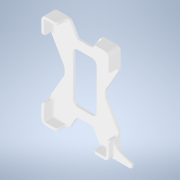
# Autodesk Inventor part: Heatpad Tray
Saved by Autodesk Inventor 2020 (Build 240168000, 168)
## iProperties
Created: 2020-02-13
Part Number: Heatpad Tray
Material: ABS Plastic
Document SubType Name: Modeling
Designer: Ishaan
Density: 1.06 g/cm^3
Appearance: Smooth - White
Author: Ishaan
Autodesk Inventor part; units mm, degrees
ref_plane "YZ Plane" through (0, 0, 0) normal (1, 0, 0) x (0, 1, 0)
sketch "Sketch1" plane through (0, 0, 0) normal (0, 0, 1) x (1, 0, 0)
  line L0 (38, -53) -> (-38, -53)
  line L1 (-38, -53) -> (-38, 53)
  line L2 (-38, 53) -> (38, 53)
  line L3 (38, 53) -> (38, -53)
  line L4 (38, -53) -> (-38, 53) construction
  line L5 (-38, -53) -> (38, 53) construction
  point P0 (0, 0)
  dimension "d0" = 76
  dimension "d1" = 106
  constraints: 12 end point, 2 midpoint, 2 parallel, 1 horizontal, 1 perpendicular
  measures "d0" distance of L1.end L2.end
  measures "d1" distance of L0.end L1.end
extrude "Extrusion1" add sketch "Sketch1" against normal blind 3
sketch "Sketch2" plane through (0, 0, 0) normal (0, 0, 1) x (1, 0, 0)
  line L0 (38, -53) -> (38, 53) projected
  line L1 (38, 53) -> (-38, 53) projected
  line L2 (-38, 53) -> (-38, -53) projected
  line L3 (-38, -53) -> (38, -53) projected
  line L4 (-35, -50) -> (-35, 50)
  line L5 (-35, 50) -> (35, 50)
  line L6 (35, 50) -> (35, -50)
  line L7 (35, -50) -> (-35, -50)
  line L8 (38, -53) -> (-38, -53) projected
  line L9 (20.5, 53) -> (-20.5, 53)
  line L10 (-20.5, 53) -> (-20.5, -53)
  line L11 (-20.5, -53) -> (20.5, -53)
  line L12 (20.5, -53) -> (20.5, 53)
  line L13 (20.5, 53) -> (-20.5, -53) construction
  line L14 (-20.5, 53) -> (20.5, -53) construction
  line L15 (-38, -53) -> (-38, 53) projected
  line L16 (38, 33) -> (-38, 33)
  line L17 (-38, 33) -> (-38, -33)
  line L18 (-38, -33) -> (38, -33)
  line L19 (38, -33) -> (38, 33)
  line L20 (38, 33) -> (-38, -33) construction
  line L21 (-38, 33) -> (38, -33) construction
  point P0 (0, 0)
  point P1 (35, -33)
  point P2 (20.5, -50)
  point P3 (20.5, -53)
  point P4 (35, 33)
  point P5 (20.5, 50)
  point P6 (-38, 33)
  point P7 (-35, 33)
  point P8 (-20.5, 50)
  point P9 (-20.5, 53)
  point P10 (-35, -33)
  point P11 (-20.5, -53)
  point P12 (-20.5, -50)
  dimension "d4" = 3
  dimension "d5" = 17.5
  dimension "d6" = 20
  constraints: 32 end point, 4 midpoint, 4 parallel, 2 horizontal, 2 perpendicular, 2 point on line, 3 other
  measures "d4" distance between parallel lines of L2 L4
  measures "d5" distance between parallel lines of L10 L2
  measures "d6" distance between parallel lines of L18 L3
extrude "Extrusion2" add sketch "Sketch2" along normal blind 11 contours L3 L12 L7 L6 L18 L0 | L16 L6 L5 L12 L1 L0 | L3 L2 L18 L4 L7 L10 | L10 L5 L4 L16 L2 L1
sketch "Sketch3" plane through (0, 0, 0) normal (0, 0, 1) x (1, 0, 0)
  line L0 (20.5, 50) -> (20.5, 53) projected
  line L1 (20.5, 53) -> (-20.5, 53) projected
  line L2 (-20.5, 53) -> (-20.5, 50) projected
  line L3 (-20.5, 50) -> (-35, 50) projected
  line L4 (-35, 50) -> (-35, 33) projected
  line L5 (-35, 33) -> (-38, 33) projected
  line L6 (-38, 33) -> (-38, -33) projected
  line L7 (-38, -33) -> (-35, -33) projected
  line L8 (-35, -33) -> (-35, -50) projected
  line L9 (-35, -50) -> (-20.5, -50) projected
  line L10 (-20.5, -50) -> (-20.5, -53) projected
  line L11 (-20.5, -53) -> (20.5, -53) projected
  line L12 (20.5, -53) -> (20.5, -50) projected
  line L13 (20.5, -50) -> (35, -50) projected
  line L14 (35, -50) -> (35, -33) projected
  line L15 (35, -33) -> (38, -33) projected
  line L16 (38, -33) -> (38, 33) projected
  line L17 (38, 33) -> (35, 33) projected
  line L18 (35, 33) -> (35, 50) projected
  line L19 (35, 50) -> (20.5, 50) projected
  line L20 (-38, 33) -> (-38, -33) projected
  line L21 (-38, -30) -> (-23, -4.0192)
  line L22 (-23, -4.0192) -> (-23, 0)
  line L23 (-20.5, -53) -> (20.5, -53) projected
  line L24 (-17.5, -53) -> (-8.8397, -38)
  line L25 (-8.8397, -38) -> (0, -38)
  line L26 (0, -38) -> (0, -53)
  line L27 (-23, 0) -> (-38, 0)
  point P0 (0, 0)
  dimension "d9" = 15
  dimension "d10" = 30
  dimension "d11" = 30
  dimension "d12" = 15
  dimension "d13" = 17.5
  constraints: 12 end point, 3 parallel, 2 midpoint, 2 perpendicular, 2 point on line
  measures "d9" distance between parallel lines of L22 L6
  measures "d10" angle of L6 L21
  measures "d11" distance of L21.start L27.end
  measures "d12" distance between parallel lines of L25 L11
  measures "d13" distance of L26.end L24.start
extrude "Extrusion3" cut sketch "Sketch3" against normal through all contours L27 L22 L21 L6 | L11 L24 L25 L26
mirror "Mirror1" about plane through (0, 0, 0) normal (1, 0, 0) of "Extrusion3"
mirror "Mirror2" about plane through (0, 0, 0) normal (0, 1, 0) of "Extrusion3", "Mirror1"
ref_plane "Work Plane1" through (0, 0, 4) normal (0, 0, -1) x (-1, 0, 0)
sketch "Sketch4" plane through (0, 0, 4) normal (0, 0, -1) x (-1, 0, 0)
  line L0 (-38, -33) -> (-35, -33) projected
  line L1 (-35, -33) -> (-35, -50) projected
  line L2 (-35, -50) -> (-20.5, -50) projected
  line L3 (-20.5, -50) -> (-20.5, -53) projected
  line L4 (-20.5, -53) -> (-38, -53) projected
  line L5 (-38, -53) -> (-38, -33) projected
  line L6 (-38, -53) -> (-17.5, -53) projected
  line L7 (-38, -53) -> (-58, -53)
  line L8 (-58, -53) -> (-58, -48)
  line L9 (-58, -48) -> (-38, -48)
  line L10 (-38, -48) -> (-38, -53)
  line L11 (-58, -48) -> (-38, -40.7206)
  line L12 (-38, -30) -> (-38, -53) projected
  line L13 (-38, -48) -> (-38, -40.7206)
  point P0 (0, 0)
  dimension "d16" = 20
  dimension "d17" = 5
  dimension "d30" = 70
  constraints: 12 end point, 2 parallel, 1 collinear, 1 horizontal, 1 perpendicular, 1 point on line
  measures "d16" distance of L8.end L9.end
  measures "d17" distance of L7.end L8.end
  measures "d30" angle of L11 L5
extrude "Extrusion4" add sketch "Sketch4" along normal mid plane 3 contours L5 L9 L11 | L5 L7 L8 L9
sketch "Sketch5" plane through (0, 0, 0) normal (0, 0, 1) x (1, 0, 0)
  line L0 (-13, -28) -> (13, -28)
  line L1 (13, -28) -> (13, 28)
  line L2 (13, 28) -> (-13, 28)
  line L3 (-13, 28) -> (-13, -28)
  line L4 (-13, -28) -> (13, 28) construction
  line L5 (13, -28) -> (-13, 28) construction
  line L6 (23, -4.0192) -> (23, 4.0192) projected
  line L7 (23, 4.0192) -> (38, 30) projected
  line L8 (38, 30) -> (38, 33) projected
  line L9 (38, 33) -> (35, 33) projected
  line L10 (35, 33) -> (35, 50) projected
  line L11 (35, 50) -> (20.5, 50) projected
  line L12 (20.5, 50) -> (20.5, 53) projected
  line L13 (20.5, 53) -> (17.5, 53) projected
  line L14 (17.5, 53) -> (8.8397, 38) projected
  line L15 (8.8397, 38) -> (-8.8397, 38) projected
  line L16 (-8.8397, 38) -> (-17.5, 53) projected
  line L17 (-17.5, 53) -> (-20.5, 53) projected
  line L18 (-20.5, 53) -> (-20.5, 50) projected
  line L19 (-20.5, 50) -> (-35, 50) projected
  line L20 (-35, 50) -> (-35, 33) projected
  line L21 (-35, 33) -> (-38, 33) projected
  line L22 (-38, 33) -> (-38, 30) projected
  line L23 (-38, 30) -> (-23, 4.0192) projected
  line L24 (-23, 4.0192) -> (-23, -4.0192) projected
  line L25 (-23, -4.0192) -> (-38, -30) projected
  line L26 (-38, -30) -> (-38, -33) projected
  line L27 (-38, -33) -> (-35, -33) projected
  line L28 (-35, -33) -> (-35, -50) projected
  line L29 (-35, -50) -> (-20.5, -50) projected
  line L30 (-20.5, -50) -> (-20.5, -53) projected
  line L31 (-20.5, -53) -> (-17.5, -53) projected
  line L32 (-17.5, -53) -> (-8.8397, -38) projected
  line L33 (-8.8397, -38) -> (8.8397, -38) projected
  line L34 (8.8397, -38) -> (17.5, -53) projected
  line L35 (17.5, -53) -> (20.5, -53) projected
  line L36 (20.5, -53) -> (20.5, -50) projected
  line L37 (20.5, -50) -> (35, -50) projected
  line L38 (35, -50) -> (35, -33) projected
  line L39 (35, -33) -> (38, -33) projected
  line L40 (38, -33) -> (38, -30) projected
  line L41 (38, -30) -> (23, -4.0192) projected
  point P0 (0, 0)
  dimension "d31" = 10
  dimension "d32" = 10
  constraints: 12 end point, 2 midpoint, 2 parallel, 1 horizontal, 1 perpendicular
  measures "d31" distance between parallel lines of L1 L6
  measures "d32" distance between parallel lines of L2 L15
extrude "Extrusion5" cut sketch "Sketch5" against normal through all contours L3 L2 L1 L0
fillet "Fillet1" radius 10 1 edges at (38, -40.7206, 4)
fillet "Fillet2" radius 2 2 edges at (58, -53, 4) (58, -48, 4)
fillet "Fillet3" radius 5 20 edges at (-17.5, -53, -1.5) (-8.8397, -38, -1.5) (17.5, -53, -1.5) (8.8397, -38, -1.5) (-17.5, 53, -1.5) (-8.8397, 38, -1.5) (8.8397, 38, -1.5) (17.5, 53, -1.5) (38, -30, -1.5) (23, -4.0192, -1.5) (23, 4.0192, -1.5) (38, 30, -1.5) (-38, -30, -1.5) (-23, -4.0192, -1.5) (-23, 4.0192, -1.5) (-38, 30, -1.5) (13, 28, -1.5) (-13, 28, -1.5) (13, -28, -1.5) (-13, -28, -1.5)
fillet "Fillet4" radius 3 16 edges at (-20.5, 51.5, 11) (-36.5, 33, 11) (-36.5, 33, 0) (-20.5, 51.5, 0) (20.5, 51.5, 11) (36.5, 33, 11) (36.5, 33, 0) (36.5, -33, 0) (36.5, -33, 11) (20.5, -51.5, 11) (20.5, -51.5, 0) (-20.5, -51.5, 0) (-20.5, -51.5, 11) (-36.5, -33, 11) (-36.5, -33, 0) (20.5, 51.5, 0)
fillet "Fillet5" radius 5 5 edges at (38, -53, 8.25) (38, -53, -0.25) (-38, -53, 4) (-38, 53, 4) (38, 53, 4)
fillet "Fillet6" radius 2 4 edges at (-35, -50, 5.5) (-35, 50, 5.5) (35, 50, 5.5) (35, -50, 5.5)
fillet "Fillet7" radius 2 20 edges at (-19, -50, 0) (-26.75, -50, 0) (-35, -31.5, 0) (-35, -40.5, 0) (-34.4142, -49.4142, 0) (-34.4142, 49.4142, 0) (-19, 50, 0) (-26.75, 50, 0) (-35, 40.5, 0) (-35, 31.5, 0) (34.4142, 49.4142, 0) (35, 40.5, 0) (35, 31.5, 0) (26.75, 50, 0) (19, 50, 0) (34.4142, -49.4142, 0) (35, -40.5, 0) (35, -31.5, 0) (26.75, -50, 0) (19, -50, 0)
fillet "Fillet8" radius 0.5 170 edges at (38, -33.8787, 10.1213) (38, -33, 5.5) (38, -32.5514, 1.4219) (37.9577, -30.6911, 0.0807) (37.6103, -29.4045, 0) (30.5, -17.0096, 0) (23.1704, -3.9736, 0) (23, 0, 0) (23.1704, 3.9736, 0) (30.5, 17.0096, 0) (37.6103, 29.4045, 0) (37.9577, 30.6911, 0.0807) (38, 32.5514, 1.4219) (38, 33, 5.5) (38, 33.8787, 10.1213) (38, 42, 11) (36.5355, 51.5355, 11) (28.25, 53, 11) (21.3787, 53, 10.1213) (20.5, 53, 5.5) (20.4716, 53, 2.5878) (19.3428, 52.8898, 0.6327) (16.6926, 51.3694, 0) (13.1699, 45.5, 0) (8.453, 38.6699, 0) (0, 38, 0) (-8.453, 38.6699, 0) (-13.1699, 45.5, 0) (-16.6926, 51.3694, 0) (-19.3428, 52.8898, 0.6327) (-20.4716, 53, 2.5878) (-20.5, 53, 5.5) (-21.3787, 53, 10.1213) (-28.25, 53, 11) (-36.5355, 51.5355, 11) (-38, 42, 11) (-38, 33.8787, 10.1213) (-38, 33, 5.5) (-38, 32.5514, 1.4219) (-37.9577, 30.6911, 0.0807) (-37.6103, 29.4045, 0) (-30.5, 17.0096, 0) (-23.1704, 3.9736, 0) (-23, 0, 0) (-23.1704, -3.9736, 0) (-30.5, -17.0096, 0) (-37.6103, -29.4045, 0) (-37.9577, -30.6911, 0.0807) (-38, -32.5514, 1.4219) (-38, -33, 5.5) (-38, -33.8787, 10.1213) (-38, -42, 11) (-36.5355, -51.5355, 11) (-28.25, -53, 11) (-21.3787, -53, 10.1213) (-20.5, -53, 5.5) (-20.4716, -53, 2.5878) (-19.3426, -52.8898, 0.6326) (-16.6926, -51.3694, 0) (-13.1699, -45.5, 0) (-8.453, -38.6699, 0) (0, -38, 0) (8.453, -38.6699, 0) (13.1699, -45.5, 0) (16.6926, -51.3694, 0) (19.3428, -52.8898, 0.6327) (20.4716, -53, 2.5878) (20.5, -53, 5.5) (21.3787, -53, 10.1213) (28.25, -53, 11) (36.5355, -51.5355, 11) (38, -42, 11) (34.4142, -49.4142, 11) (28.25, -50, 11) (21.3787, -50, 10.1213) (20.5, -50, 5.5) (20.4568, -50, 2.4927) (35, -33.8787, 10.1213) (35, -33, 5.5) (35, -32.9568, 2.4927) (35, -42, 11) (-28.25, -50, 11) (-34.4142, -49.4142, 11) (-35, -42, 11) (-35, -33.8787, 10.1213) (-35, -33, 5.5) (-35, -32.9568, 2.4927) (-34.2327, -31.5394, 0.4251) (-20.5, -50, 5.5) (-20.4568, -50, 2.4927) (-19.0394, -49.2327, 0.4251) (-21.3787, -50, 10.1213) (-35, 42, 11) (-34.4142, 49.4142, 11) (-28.25, 50, 11) (-21.3787, 50, 10.1213) (-20.5, 50, 5.5) (-20.4568, 50, 2.4927) (-19.0394, 49.2327, 0.4251) (-35, 33, 5.5) (-35, 32.9568, 2.4927) (-34.2327, 31.5394, 0.4251) (-35, 33.8787, 10.1213) (21.3787, 50, 10.1213) (28.25, 50, 11) (34.4142, 49.4142, 11) (35, 42, 11) (35, 33.8787, 10.1213) (35, 33, 5.5) (35, 32.9568, 2.4927) (34.2327, 31.5394, 0.4251) (20.4568, 50, 2.4927) (19.0394, 49.2327, 0.4251) (20.5, 50, 5.5) (-13.1699, 45.5, -3) (-17.8868, 52.3301, -3) (-26.6934, 53, -3) (-36.5355, 51.5355, -3) (-38, 39.6699, -3) (-37.8296, 30.0457, -3) (-30.5, 17.0096, -3) (-23.1704, 3.9736, -3) (-23, 0, -3) (-23.1704, -3.9736, -3) (-30.5, -17.0096, -3) (-37.8296, -30.0457, -3) (-38, -39.6699, -3) (-36.5355, -51.5355, -3) (-26.6934, -53, -3) (-17.8868, -52.3301, -3) (-13.1699, -45.5, -3) (-8.453, -38.6699, -3) (0, -38, -3) (8.453, -38.6699, -3) (13.1699, -45.5, -3) (17.8868, -52.3301, -3) (26.6934, -53, -3) (36.5355, -51.5355, -3) (38, -39.6699, -3) (37.8296, -30.0457, -3) (30.5, -17.0096, -3) (23.1704, -3.9736, -3) (23, 0, -3) (23.1704, 3.9736, -3) (30.5, 17.0096, -3) (37.8296, 30.0457, -3) (38, 39.6699, -3) (36.5355, 51.5355, -3) (26.6934, 53, -3) (17.8868, 52.3301, -3) (13.1699, 45.5, -3) (8.453, 38.6699, -3) (0, 38, -3) (-8.453, 38.6699, -3) (13, 0, -3) (11.5355, -26.5355, -3) (0, -28, -3) (-11.5355, -26.5355, -3) (-13, 0, -3) (-11.5355, 26.5355, -3) (0, 28, -3) (11.5355, 26.5355, -3) (0, 28, 0) (-11.5355, 26.5355, 0) (-13, 0, 0) (-11.5355, -26.5355, 0) (0, -28, 0) (11.5355, -26.5355, 0) (13, 0, 0) (11.5355, 26.5355, 0)
fillet "Fillet9" radius 1 6 edges at (38, -37.2196, 5.5) (38, -44.3603, 5.5) (36.5355, -51.5355, 5.5) (38, -44.3603, 2.5) (38, -37.2196, 2.5) (36.5355, -51.5355, 2.5)
fillet "Fillet10" radius 1 8 edges at (57.4142, -52.4142, 5.5) (58, -50.2002, 5.5) (34.63, -53, 5.8285) (46.1583, -53, 5.5) (58, -50.2002, 2.5) (57.4142, -52.4142, 2.5) (46.1583, -53, 2.5) (34.63, -53, 2.1715)
ref_plane "Work Plane2" through (0, 0, 4) normal (0, 0, 1) x (1, 0, 0)
body "Solid1"
